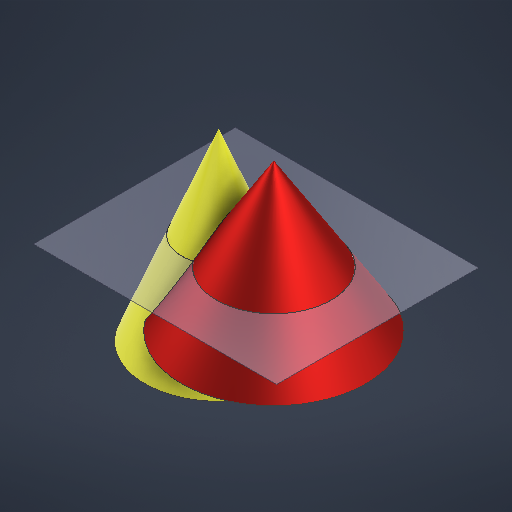
# Autodesk Inventor part: Пересечение поверхностей
Saved by Autodesk Inventor 2026 (Build 300175000, 175)
## iProperties
Created: 2025-11-23
Part Number: Пересечение поверхностей
Material: Типовые
Document SubType Name: Modeling
Designer: nittle
Density: 1 g/cm^3
Appearance: По умолчанию
Mass: 326.954 g
Surface Area: 325.726 cm^2
Volume: 326.954 cm^3
Author: nittle
Autodesk Inventor part; units mm, degrees
ref_plane "YZ Plane" through (0, 0, 0) normal (1, 0, 0) x (0, 1, 0)
ref_plane "XY Plane" through (0, 0, 0) normal (0, 0, 1) x (1, 0, 0)
sketch "Эскиз2" plane through (0, 0, 0) normal (0, 0, 1) x (1, 0, 0)
  line L0 (0, 0) -> (40, 0)
  line L1 (0, 0) -> (-40, 0)
  line L2 (0, 100) -> (-40, 0)
  line L3 (0, 100) -> (40, 0)
  line L4 (0, 100) -> (0, 0)
  dimension "d0" = 40
  dimension "d1" = 40
  dimension "d2" = 100
  constraints: 10 end point, 2 horizontal, 1 perpendicular
  measures "d0" distance of L0.start L0.end
  measures "d1" distance of L0.start L1.end
  measures "d2" distance of L0.start L2.start
revolve "Вращение1" add sketch "Эскиз2" angle 360 about axis through (0, 100, 0) along (0, -1, 0) contours L1 L2 L4
sketch "Эскиз3" plane through (0, 0, 0) normal (0, 0, 1) x (1, 0, 0)
  line L0 (-40, 0) -> (40, 0) projected
  line L1 (0, 0) -> (30, 0)
  line L2 (30, 0) -> (30, 20)
  line L3 (30, 20) -> (80, 20)
  line L4 (30, 20) -> (-20, 20)
  line L5 (30, 20) -> (30, 100)
  line L6 (30, 100) -> (80, 20)
  line L7 (30, 100) -> (-20, 20)
  point P0 (0, 100)
  dimension "d4" = 30
  dimension "d5" = 20
  dimension "d6" = 50
  dimension "d7" = 50
  dimension "d8" = 80
  constraints: 14 end point, 2 horizontal, 1 perpendicular, 1 point on line, 1 vertical
  measures "d4" distance of L1.start L1.end
  measures "d5" distance of L1.end L2.end
  measures "d6" distance of L2.end L3.end
  measures "d7" distance of L2.end L4.end
  measures "d8" distance of L2.end L5.end
revolve "Вращение2" add sketch "Эскиз3" angle 360 about axis through (30, 20, 0) along (0, 1, 0) contours L5 L6 L3
ref_plane "РабПлоскость1" through (0, 50, 0) normal (0, 1, 0) x (-1, 0, 0)
sketch "Эскиз5" plane through (0, 50, 0) normal (0, 1, 0) x (-1, 0, 0)
  line L0 (-86.1125, -55.112) -> (-86.1125, 54.6369)
  line L1 (-86.1125, 54.6369) -> (45.9663, 54.6369)
  line L2 (45.9663, 54.6369) -> (45.9663, -55.112)
  line L3 (45.9663, -55.112) -> (-86.1125, -55.112)
  circle A0 centre (0, 0) radius 40 projected
  arc A1 (9.6, 30.5261) -> (9.6, -30.5261) centre (-30, 0) ccw projected
  arc A2 (9.6, 30.5261) -> (9.6, -30.5261) centre (0, 0) ccw projected
  circle A3 centre (0, 0) radius 40 projected
  constraints: 8 end point, 3 perpendicular, 2 vertical alignment, 1 vertical
extrude "Выдавливание2" add sketch "Эскиз5" along normal blind 0.1 separate body contours L0 L1 L2 L3 | A0 A1 A2 | A1 A2 A0 | A0 A1
split body "Разделение1" result two bodies by plane through (0, 50, 0) normal (0, 1, 0) bodies 1 first body at (16.8095, 67.609, -14.5712)
